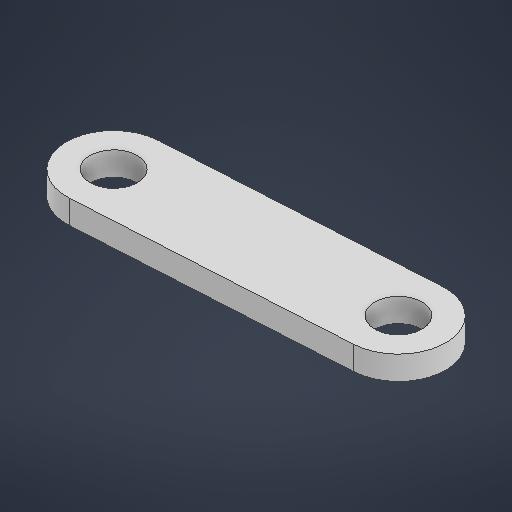
# Autodesk Inventor part: Aparatus_Connector
Saved by Autodesk Inventor 2026.2 (Build 302298000, 298)
## iProperties
Created: 2025-12-30
Part Number: Aparatus_Connector
Material: Generic
Document SubType Name: Modeling
Designer: Cobble
Density: 1 g/cm^3
Appearance: Default
Author: Cobble
Autodesk Inventor part; units mm, degrees
ref_plane "YZ Plane" through (0, 0, 0) normal (1, 0, 0) x (0, 1, 0)
ref_plane "XZ Plane" through (0, 0, 0) normal (0, 1, 0) x (-1, 0, 0)
ref_plane "XY Plane" through (0, 0, 0) normal (0, 0, 1) x (1, 0, 0)
sketch "Sketch1" plane through (0, 0, 0) normal (0, 0, 1) x (1, 0, 0)
  circle A0 centre (0, 0) radius 93.188 construction
  line L0 (0, 0) -> (-85.0386, 38.1109) construction
  line L1 (0, 0) -> (93.188, 0) construction
  circle A1 centre (-85.0386, 38.1109) radius 4
  circle A2 centre (0, 0) radius 60 construction
  arc A3 (-39.5143, 40.7395) -> (-85.0386, 38.1109) centre (-60, 0) ccw construction
  line L2 (-60, 0) -> (-39.5143, 40.7395) construction
  line L3 (-60, 0) -> (-85.0386, 38.1109) construction
  circle A4 centre (-39.5143, 40.7395) radius 4
  circle A5 centre (-85.0386, 38.1109) radius 8
  circle A6 centre (-39.5143, 40.7395) radius 8
  line L4 (-84.5774, 30.1242) -> (-39.0532, 32.7528)
  line L5 (-39.9755, 48.7262) -> (-85.4998, 46.0976)
  dimension "d3" = 120
  dimension "d0" = 186.376
  dimension "d1" = 155.86
  dimension "d2" = 8
  dimension "d4" = 60
  dimension "d5" = 8
  dimension "d6" = 16
  dimension "d7" = 16
  dimension "d8" = 60
  dimension "d9" = 40.7395
  dimension "d10" = 39.5143
  constraints: 12 end point, 8 point on circle, 6 centre point, 6 coincident, 4 tangent, 1 equal length, 1 horizontal, 1 horizontal alignment, 2 other
  measures "d0" diameter of A0
  measures "d1" angle of L1 L0
  measures "d2" diameter of A1
  measures "d4" angle of L2 L3
  measures "d5" diameter of A4
  measures "d6" diameter of A5
  measures "d7" diameter of A6
  measures "d8" distance of point (0, 0) L2.start
  measures "d9" vertical distance of point (0, 0) L2.end
  measures "d10" horizontal distance of point (0, 0) L2.end
extrude "Extrusion1" add sketch "Sketch1" along normal blind 4
body "Solid1"
